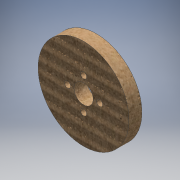
# Autodesk Inventor part: CouplingHead
Saved by Autodesk Inventor 2016 (Build 200138000, 138)
## iProperties
Created: 2015-11-25
Part Number: CouplingHead
Material: MDF Medium Density Fiberboard
Document SubType Name: Modeling
Designer: momem
Density: 0.8 g/cm^3
Appearance: Cardboard - Corrugated
MotorCouplingScrewDiameter: 3.000 mm
MotorCouplingScrewDistance: 7.938 mm
d0: 45.078 mm
d3: 4.000 ul
d5: 360.00 deg
d7: 9.525 mm
BearingDiameter: 24.000 mm
WoodThickness: 6.390 mm
BearingWidth: 7.000 mm
BearingShaftDiameter: 8.000 mm
ZipTieWidth: 2.500 mm
ZipTieThickness: 1.100 mm
ZipTieClearance: 1.000 mm
ZipTieDistance: 10.000 mm
BearingHolderHeight: 13.100 mm
d8: 6.390 mm
d9: 0.00 deg
MotorWidth: 37.000 mm
SupportClearance: 5.000 mm
MotorShaftWidth: 12.000 mm
CouplingWidth: 0.375 in
CouplingDiameter: 0.870 in
DiskGap: 75.835 mm
d28: 360.00 deg
MotorWheel: 45.078 mm
Author: momem
Autodesk Inventor part; units mm, degrees
ref_plane "YZ Plane" through (0, 0, 0) normal (1, 0, 0) x (0, 1, 0)
ref_plane "XZ Plane" through (0, 0, 0) normal (0, 1, 0) x (-1, 0, 0)
ref_plane "XY Plane" through (0, 0, 0) normal (0, 0, 1) x (1, 0, 0)
sketch "Sketch1" plane through (0, 0, 0) normal (0, 1, 0) x (-1, 0, 0)
  circle A0 centre (0, 0) radius 22.539
  circle A1 centre (7.9375, 0) radius 1.5
  circle A2 centre (0, 7.9375) radius 1.5
  circle A3 centre (-7.9375, 0) radius 1.5
  circle A4 centre (0, -7.9375) radius 1.5
  circle A5 centre (0, 0) radius 4.7625
  dimension "d0" = 45.078
  dimension "MotorCouplingScrewDiameter" = 3
  dimension "MotorCouplingScrewDistance" = 7.9375
  dimension "d5" = 360
  dimension "d7" = 9.525
  constraints: 6 centre point, 2 coincident, 1 horizontal alignment, 9 other
  measures "d0" diameter of A0
  measures "MotorCouplingScrewDiameter" diameter of A1
  measures "MotorCouplingScrewDistance" distance of point (0, 0) A1.centre
  measures "d7" diameter of A5
extrude "Extrusion1" add sketch "Sketch1" along normal blind 6.39
equation "\"d0\" = MotorWheel"
equation "\"d8\" = WoodThickness"
equation "\"BearingHolderHeight\" = 13.1"
equation "\"MotorWheel\" = 45.078"
equation "\"WoodThickness\" = 6.39"
body "Solid1"
